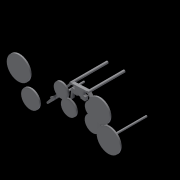
# Autodesk Inventor part: Drums
Saved by Autodesk Inventor 2020 (Build 240168000, 168)
## iProperties
Created: 2020-04-10
Part Number: Drums
Material: Generic
Document SubType Name: Modeling
Designer: valer
Density: 1 g/cm^3
Appearance: Default
Author: valer
Autodesk Inventor part; units mm, degrees
ref_plane "YZ Plane" through (0, 0, 0) normal (1, 0, 0) x (0, 1, 0)
ref_plane "XZ Plane" through (0, 0, 0) normal (0, 1, 0) x (-1, 0, 0)
sketch "Sketch1" plane through (0, 0, 0) normal (0, 0, 1) x (1, 0, 0)
  line L0 (-40.3555, 383.4313) -> (111.0673, 366.2011)
  line L1 (111.0673, 366.2011) -> (102.4522, 290.4897)
  line L2 (102.4522, 290.4897) -> (-48.9706, 307.7199)
  line L3 (-48.9706, 307.7199) -> (-40.3555, 383.4313)
  line L4 (-87.7484, 312.1324) -> (140.3854, 286.1733)
  line L5 (140.3854, 286.1733) -> (132.8088, 219.5891)
  line L6 (132.8088, 219.5891) -> (-95.3249, 245.5482)
  line L7 (-95.3249, 245.5482) -> (-87.7484, 312.1324)
  circle A0 centre (175.3182, 379.203) radius 20.5535
  circle A1 centre (-115.4076, 365.5218) radius 21.0224
  circle A2 centre (558.8, -101.6) radius 15.2961
  circle A3 centre (-514.4431, -124.7218) radius 14.6004
  line L8 (-128.6785, 349.2176) -> (-505.2263, -113.3983) construction
  line L9 (-94.4085, 366.51) -> (154.7875, 378.2368) construction
  line L10 (187.1074, 362.3667) -> (548.0677, -90.701) construction
  line L11 (-87.7484, 312.1324) -> (-107.085, 142.1977)
  circle A4 centre (-732.6645, 423.8625) radius 24.2389
  circle A5 centre (-732.6645, 423.8625) radius 201.0267
  circle A6 centre (649.2875, 481.0125) radius 192.9655
  circle A7 centre (816.1948, 122.9166) radius 202.4756
  circle A8 centre (-122.1817, 9.525) radius 133.5288
  circle A9 centre (-529.0436, 65.0875) radius 157.5724
  circle A10 centre (-255.7105, 206.375) radius 123.1837
  circle A11 centre (275.6471, 184.2457) radius 119.3572
  circle A12 centre (291.6085, -20.9726) radius 137.6551
  line L12 (-519.4107, -110.9924) -> (-135.7782, 360.3274)
  line L13 (-99.1269, 378.8214) -> (158.4473, 390.9425)
  line L14 (194.9233, 373.0316) -> (560.0295, -86.3534)
  line L15 (-500.0898, -127.3963) -> (-115.9822, 344.5072)
  line L16 (-98.1626, 353.4988) -> (159.8736, 365.6417)
  line L17 (174.0312, 358.6899) -> (544.8706, -107.9199)
  line L18 (-74.6538, 313.5326) -> (-94.3852, 140.1286)
  line L19 (-100.0538, 313.5326) -> (-119.4555, 143.026)
  line L20 (-100.0538, 313.5326) -> (-74.6538, 313.5326)
  line L21 (0, 255.1359) -> (53.975, 248.9942)
  line L22 (53.975, 248.9942) -> (36.2304, 93.0509)
  line L23 (36.2304, 93.0509) -> (-17.7446, 99.1926)
  line L24 (-17.7446, 99.1926) -> (0, 255.1359)
  line L25 (-444.5, 9.525) -> (-390.525, 47.3529)
  line L26 (-390.525, 47.3529) -> (-276.9226, -114.7417)
  line L27 (-276.9226, -114.7417) -> (-330.8976, -152.5695)
  line L28 (-330.8976, -152.5695) -> (-444.5, 9.525)
  point P0 (0, 0)
  point P1 (353.9374, 101.7631)
  point P2 (359.158, 98.9691)
  point P3 (370.3781, 111.6358)
  point P4 (-43.4686, 356.0727)
  point P5 (-74.9784, 310.6793)
  point P6 (-82.555, 244.0951)
  point P7 (-2.2955, 234.9625)
  point P8 (51.6795, 228.8208)
  point P9 (110.7406, 363.3296)
  point P10 (-28.89, 382.1267)
  point P11 (-40.5665, 381.5772)
  point P12 (-376.9531, 23.8858)
  point P13 (-376.1743, 26.8765)
  point P14 (-375.4084, 25.7836)
  point P15 (206.3261, 87.0822)
  point P16 (-231.992, 85.4963)
  point P17 (-152.1677, 139.6434)
  point P18 (-433.7732, -5.7806)
  point P19 (-502.5158, -90.2359)
  point P20 (-371.569, 70.6416)
  point P21 (384.2743, 134.7858)
  point P22 (226.299, 292.9237)
  point P23 (251.9859, 301.2341)
  dimension "d0" = 152.4
  dimension "d1" = 76.2
  dimension "d2" = 12.5196
  dimension "d3" = 12.8203
  dimension "d4" = 12.8523
  dimension "d5" = 12.3848
  dimension "d15" = 30.5921
  constraints: 58 end point, 21 point on circle, 13 centre point, 11 parallel, 4 perpendicular, 3 collinear, 1 coincident, 1 horizontal, 1 point on line
  measures "d0" distance of L0.start L0.end
  measures "d1" distance of L2.end L0.start
  measures "d2" distance between parallel lines of L8 L12
  measures "d3" distance between parallel lines of L8 L15
  measures "d4" distance between parallel lines of L11 L18
  measures "d5" distance between parallel lines of L11 L19
  measures "d15" diameter of A2
extrude "Extrusion1" add sketch "Sketch1" against normal blind 635 contours A0 | A1 | A2 | A3
extrude "Extrusion2" add sketch "Sketch1" against normal blind 50.8 contours L0 L13 L3 | L13 A0 L16 L1 L0 | L0 L1 L16 L3 L13 | L3 L16 A1 L13 | L16 L1 L2 L3 | L2 L4 L5 L6 L22 L21 L24 L18 | A1 L15 A10 L12 | L14 A11 L17 A0 | L18 L6 L7 L4 | L4 L7 L11 A8 L19 L20 L18 | A10 L15 L12 | L18 A8 L11 L6 | A10 L15 L26 A9 L12 | L14 A2 L17 A11 | A11 A12 | A9 L26 L12 | L12 L28 L15 A9 | A9 L15 A3 L12 | L26 A9 L15 L28 L12 picked at (299.5607, -83.2426)
extrude "Extrusion3" add sketch "Sketch1" along normal blind 25.4 contours L12 A10 | A10 L15 L12 | L14 A11 L17 | A11 L14 | L17 A11 A12 | A10 A8 L15 | A12 A11 | A11 A12 | A8 A10 | A9 L26 L12 | A10 A8 | L15 A9 L26 | L12 L28 L15 A9 | L26 A9 L15 L28 L12 | L12 L28 L25 | A9 L28 L15 | L15 L28 A9
ref_plane "Work Plane1" through (0, 0, 254) normal (0, 0, 1) x (1, 0, 0)
sketch "Sketch2" plane through (0, 0, 254) normal (0, 0, 1) x (1, 0, 0)
  circle A0 centre (-732.6645, 423.8625) radius 201.0267 projected
  circle A1 centre (649.2875, 481.0125) radius 192.9655 projected
  circle A2 centre (816.1948, 122.9166) radius 202.4756 projected
  circle A3 centre (-529.0436, 65.0875) radius 157.5724 projected
  point P0 (0, 0)
extrude "Extrusion4" add sketch "Sketch2" along normal blind 25.4
body "Solid1"
